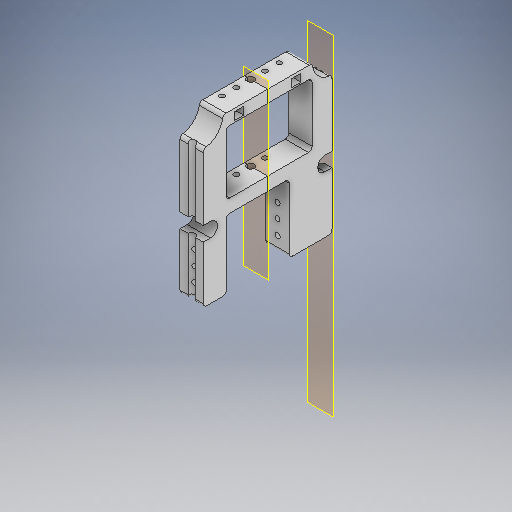
# Autodesk Inventor part: OdomPod
Saved by Autodesk Inventor 2026.1 (Build 301233000, 233)
## iProperties
Created: 2025-10-05
Part Number: OdomPod
Material: Generic
Document SubType Name: Modeling
Designer: Teddy
Density: 1 g/cm^3
Appearance: Default
Author: Teddy
Autodesk Inventor part; units mm, degrees
ref_plane "YZ Plane" through (0, 0, 0) normal (1, 0, 0) x (0, 1, 0)
ref_plane "XZ Plane" through (0, 0, 0) normal (0, 1, 0) x (-1, 0, 0)
ref_plane "Work Plane1" through (0, 0, 0) normal (0, 0, 1) x (1, 0, 0)
sketch "Sketch1" plane through (0, 0, 0) normal (0, 0, 1) x (1, 0, 0)
  circle A0 centre (0, 120.65) radius 2.1844 projected
  circle A1 centre (0, 31.75) radius 2.1844 projected
  circle A2 centre (0, 6.35) radius 2.1844 projected
  line L0 (1.8034, -21.3614) -> (-1.8034, -21.3614) projected
  line L1 (10.3187, 133.35) -> (-10.3187, 133.35)
  line L2 (-10.3187, 133.35) -> (-10.3187, -21.3614)
  line L3 (-10.3187, -21.3614) -> (10.3187, -21.3614)
  line L4 (10.3187, -21.3614) -> (10.3187, 133.35)
  line L5 (-10.3187, 133.35) -> (-10.3187, 71.0917) projected
  line L6 (10.3187, 71.0917) -> (10.3187, 133.35) projected
  point P0 (0, 0)
  constraints: 8 end point, 2 parallel, 1 horizontal, 1 horizontal alignment, 1 perpendicular
ref_plane "Work Plane2" through (-10.3188, -133.35, 114.3) normal (0, 0, -1) x (0, 1, 0)
extrude "Extrusion1" add sketch "Sketch1" along normal up to surface (114.3 mm away) contours A0 | A1 | A2 | L0 L3 L2 L1 L4
sketch "Sketch2" plane through (-10.3187, -21.3614, 0) normal (-1, 0, 0) x (0, 0, 1)
  line L0 (0, 0) -> (114.3, 0) projected
  line L1 (38.0439, 0) -> (93.9239, 0)
  line L2 (93.9239, 0) -> (93.9239, 76.2)
  line L3 (93.9239, 76.2) -> (38.0439, 76.2)
  line L4 (38.0439, 76.2) -> (38.0439, 0)
  line L5 (17.7239, 143.8065) -> (93.9239, 143.8065)
  line L6 (93.9239, 143.8065) -> (93.9239, 87.9265)
  line L7 (93.9239, 87.9265) -> (17.7239, 87.9265)
  line L8 (17.7239, 87.9265) -> (17.7239, 143.8065)
  line L9 (114.3, 0) -> (114.3, 154.7114) projected
  circle A0 centre (114.3, 154.7114) radius 17.3589
  line L10 (0, 0) -> (0, 154.7114) projected
  circle A1 centre (0, 154.7114) radius 17.3589
  point P0 (0, 21.3614)
  point P1 (93.9239, 0)
  dimension "d2" = 76.2
  dimension "d3" = 55.88
  dimension "d4" = 55.88
  dimension "d5" = 76.2
  constraints: 16 end point, 4 parallel, 2 centre point, 2 horizontal, 2 perpendicular, 2 point on line, 1 equal radius
  measures "d2" distance of L1.end L2.end
  measures "d3" distance between parallel lines of L2 L4
  measures "d4" distance between parallel lines of L5 L7
  measures "d5" distance of L5.start L5.end
extrude "Extrusion2" cut sketch "Sketch2" against normal blind 25.4
sketch "Sketch3" plane through (-10.3187, 133.35, 17.3589) normal (0, 1, 0) x (1, 0, 0)
  circle A0 centre (5.5562, -39.7911) radius 3.175 projected
  circle A1 centre (5.5562, -27.0911) radius 2.286
  circle A2 centre (5.5562, -52.4911) radius 2.286
  point P0 (10.3187, 17.3589)
  dimension "d10" = 4.572
  dimension "d11" = 12.7
  dimension "d12" = 12.7
  constraints: 2 centre point, 2 vertical alignment, 1 equal radius
  measures "d10" diameter of A1
  measures "d11" distance of A0.centre A1.centre
  measures "d12" distance of A0.centre A2.centre
extrude "Extrusion3" cut sketch "Sketch3" against normal blind 127
sketch "Sketch4" plane through (-10.3187, -21.3614, 38.0439) normal (0, 0, 1) x (1, 0, 0)
  circle A0 centre (10.3187, 40.4114) radius 2.1844 projected
  circle A1 centre (10.3187, 27.7114) radius 2.286
  circle A2 centre (10.3187, 53.1114) radius 2.286
  point P0 (10.3187, 21.3614)
  dimension "d20" = 4.572
  dimension "d21" = 12.7
  dimension "d22" = 12.7
  constraints: 2 centre point, 1 equal radius
  measures "d20" diameter of A2
  measures "d21" distance of A0.centre A2.centre
  measures "d22" distance of A1.centre A0.centre
extrude "Extrusion4" cut sketch "Sketch4" along normal through all both and the other way through all
fillet "Fillet1" radius 3.175 14 edges at (0, 115.9911, 0) (0, 133.35, 17.3589) (0, 122.4451, 17.7239) (0, 66.5651, 17.7239) (0, 66.5651, 93.9239) (0, 122.4451, 93.9239) (0, 133.35, 96.9411) (0, 115.9911, 114.3) (0, 54.8386, 93.9239) (0, 54.8386, 38.0439) (0, -21.3614, 38.0439) (0, -21.3614, 93.9239) (0, -21.3614, 114.3) (0, -21.3614, 0)
sketch "Sketch5" plane through (-10.3187, -21.3614, 111.125) normal (0, -1, 0) x (1, 0, 0)
  circle A0 centre (10.3187, -111.125) radius 3.175
  line L0 (20.6375, -107.95) -> (0, -107.95) projected
  line L1 (8.1343, 3.175) -> (12.5031, 3.175) projected
  circle A1 centre (10.3187, 3.175) radius 3.175
  constraints: 2 centre point, 1 coincident, 1 midpoint, 1 tangent
extrude "Extrusion5" cut sketch "Sketch5" along normal through all both and the other way through all
sketch "Sketch6" plane through (-10.3187, -18.1864, 0) normal (-1, 0, 0) x (0, 0, 1)
  line L0 (35.941, 148.9964) -> (27.559, 148.9964)
  line L1 (27.559, 148.9964) -> (27.559, 142.1384)
  line L2 (27.559, 142.1384) -> (35.941, 142.1384)
  line L3 (35.941, 142.1384) -> (35.941, 148.9964)
  line L4 (20.287, 151.5364) -> (94.013, 151.5364) projected
  line L5 (29.6672, 144.1958) -> (29.6672, 156.2989) construction
  line L6 (33.8328, 144.1958) -> (33.8328, 156.2989) construction
  line L7 (29.6672, 144.1958) -> (33.8328, 144.1958) construction
  line L8 (31.75, 144.1958) -> (31.75, 158.4124) construction
  line L9 (80.4672, 144.1958) -> (80.4672, 156.2989) construction
  line L10 (84.6328, 144.1958) -> (84.6328, 156.2989) construction
  line L11 (80.4672, 144.1958) -> (84.6328, 144.1958) construction
  line L12 (82.55, 144.1958) -> (82.55, 159.5475) construction
  line L13 (78.359, 142.1384) -> (86.741, 142.1384)
  line L14 (86.741, 142.1384) -> (86.741, 148.9964)
  line L15 (86.741, 148.9964) -> (78.359, 148.9964)
  line L16 (78.359, 148.9964) -> (78.359, 142.1384)
  point P0 (0, 18.1864)
  point P1 (86.741, 145.5674)
  point P2 (78.359, 145.5674)
  dimension "d23" = 8.382
  dimension "d24" = 6.858
  dimension "d25" = 2.54
  dimension "d26" = 2.54
  dimension "d27" = 8.382
  dimension "d28" = 6.858
  constraints: 32 end point, 6 vertical, 4 midpoint, 4 parallel, 3 horizontal, 3 perpendicular, 10 other
  measures "d23" distance of L0.start L0.end
  measures "d24" distance of L2.end L0.start
  measures "d25" distance between parallel lines of L4 L0
  measures "d26" distance between parallel lines of L4 L15
  measures "d27" distance of point (86.741, 145.567) point (78.359, 145.567)
  measures "d28" distance of L15.end L13.start
extrude "Extrusion6" cut sketch "Sketch6" against normal blind 25.4
sketch "Sketch7" plane through (-10.3187, 133.35, 94.013) normal (0, 1, 0) x (1, 0, 0)
  circle A0 centre (5.5563, 11.463) radius 2.0828 projected
  circle A1 centre (5.5563, 62.263) radius 2.0828 projected
  point P0 (10.3187, 94.013)
extrude "Extrusion7" cut sketch "Sketch7" against normal blind 25.4
sketch "Sketch8" plane through (-10.3187, -18.1864, 0) normal (-1, 0, 0) x (0, 0, 1)
  circle A0 centre (6.35, 5.4864) radius 1.4859 projected
  line L0 (6.35, 69.4596) -> (6.35, 72.4314) projected
  circle A1 centre (6.35, 68.9864) radius 1.4859 projected
  circle A2 centre (107.95, 5.4864) radius 1.4859 projected
  circle A3 centre (107.95, 68.9864) radius 1.4859 projected
  line L1 (114.3, 0) -> (114.3, 131.2494) projected
  line L2 (114.3, 12.1752) -> (0, 12.1752)
  line L3 (0, 0) -> (0, 131.2494) projected
  line L4 (0, 12.1752) -> (0, -5.3877)
  line L5 (0, -5.3877) -> (114.3, -5.3877)
  line L6 (114.3, -5.3877) -> (114.3, 12.1752)
  circle A4 centre (107.95, 68.9864) radius 6.35
  line L7 (107.95, 62.6364) -> (114.3, 62.6364)
  line L8 (107.95, 75.3364) -> (114.3, 75.3364)
  circle A5 centre (6.35, 68.9864) radius 6.35
  line L9 (6.35, 62.6364) -> (0, 62.6364)
  line L10 (6.35, 75.3364) -> (0, 75.3364)
  line L11 (0, 62.6364) -> (0, 75.3364)
  line L12 (114.3, 62.6364) -> (114.3, 75.3364)
  point P0 (0, 18.1864)
  constraints: 20 end point, 6 perpendicular, 6 point on line, 6 tangent, 4 point on circle, 2 centre point, 2 coincident, 2 collinear, 1 horizontal, 1 vertical
extrude "Extrusion8" cut sketch "Sketch8" against normal blind 25.4 contours A0 | A1 | A2 | A3 | L6 L5 L4 L3 L2 L1 | L7 A4 L1 | A4 L8 L1 | A4 | L3 A5 L9 | L3 L10 A5 | A5
fillet "Fillet2" radius 3.175 8 edges at (-6.7469, -6.0112, 0) (6.7469, -6.0112, 0) (0, -6.0112, 3.175) (0, -6.0112, 38.0439) (6.7469, -6.0112, 114.3) (0, -6.0112, 111.125) (-6.7469, -6.0112, 114.3) (0, -6.0112, 93.9239)
ref_plane "Work Plane3" through (-10.3187, 44.45, 57.15) normal (0, 0, 1) x (1, 0, 0)
split body "Split1" result two bodies by plane through (-10.3187, 44.45, 57.15) normal (0, 0, 1) first body at (-9.8187, 79.9844, 107.508)
body "Solid2"
body "Solid3"
